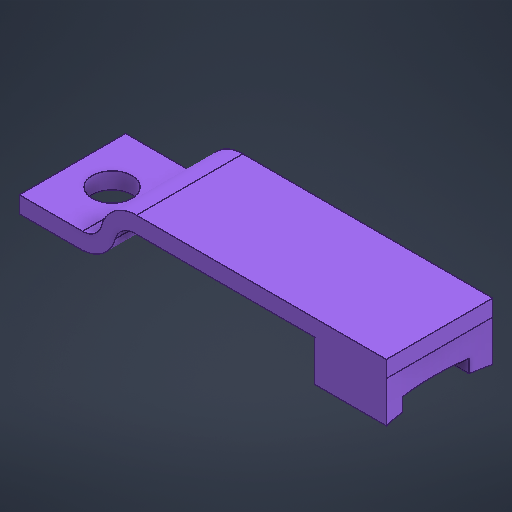
# Autodesk Inventor part: measuring_support1
Saved by Autodesk Inventor 2026.1 (Build 301233000, 233)
## iProperties
Created: 2026-01-06
Part Number: measuring_support1
Material: Generic
Document SubType Name: Modeling
Designer: emanuel
Density: 1 g/cm^3
Appearance: Violet
Author: emanuel
Autodesk Inventor part; units mm, degrees
ref_plane "YZ Plane" through (0, 0, 0) normal (1, 0, 0) x (0, 1, 0)
ref_plane "XZ Plane" through (0, 0, 0) normal (0, 1, 0) x (-1, 0, 0)
ref_plane "XY Plane" through (0, 0, 0) normal (0, 0, 1) x (1, 0, 0)
sketch "Sketch1" plane through (0, 0, 0) normal (0, 1, 0) x (-1, 0, 0)
  circle A0 centre (0, 0) radius 39.95
  circle A1 centre (0, 0) radius 35.05
  line L0 (0, 0) -> (0, -5.05)
  line L1 (0, -5.05) -> (60, -5.05)
  line L2 (60, -5.05) -> (60, 5.05)
  line L3 (60, 5.05) -> (0, 5.05)
  line L4 (0, 5.05) -> (0, -5.05)
  line L5 (0, -5.05) -> (60, -5.05)
  line L6 (60, -5.05) -> (60, -8.05)
  line L7 (60, -8.05) -> (0, -8.05)
  line L8 (0, -8.05) -> (0, -5.05)
  line L9 (0, 5.05) -> (60, 5.05)
  line L10 (60, 5.05) -> (60, 8.05)
  line L11 (60, 8.05) -> (0, 8.05)
  line L12 (0, 8.05) -> (0, 5.05)
  line L13 (39.95, 0) -> (44.95, 0)
  line L14 (44.95, 0) -> (44.95, -8.05)
  line L15 (44.95, 0) -> (44.95, 8.05)
  point P0 (34.113, 8.05)
  point P1 (34.113, -8.05)
  point P2 (44.95, -5.05)
  point P3 (34.6843, -5.05)
  point P4 (34.6843, 5.05)
  point P5 (44.95, 5.05)
  point P6 (39.6295, 5.05)
  point P7 (39.6295, -5.05)
  dimension "d0" = 79.9
  dimension "d1" = 70.1
  dimension "d2" = 5.05
  dimension "d3" = 60
  dimension "d4" = 10.1
  dimension "d5" = 60
  dimension "d6" = 3
  dimension "d7" = 60
  dimension "d8" = 3
  dimension "d9" = 5
  constraints: 32 end point, 6 parallel, 4 horizontal, 4 perpendicular, 3 point on line, 2 coincident, 1 centre point, 1 vertical, 3 other
  measures "d1" diameter of A1
  measures "d2" distance of L0.start L0.end
  measures "d3" distance of L3.end L2.end
  measures "d4" distance of L2.end L1.end
  measures "d5" distance of L6.end L7.end
  measures "d6" distance of L5.end L6.end
  measures "d7" distance of L11.end L10.end
  measures "d8" distance of L10.end L9.end
  measures "d9" distance of L13.start L13.end
extrude "Extrusion1" add sketch "Sketch1" along normal blind 4.2 contours A0 L1 A1 L3 | L13 L14 L1 A0 | A0 L3 L15 L13 | L3 A1 L11 A0 | A0 L11 L15 L3 | L1 L14 L7 A0 | A0 L7 A1 L1
extrude "Extrusion2" add sketch "Sketch1" against normal blind 2 contours L3 A1 L11 A0 | A0 L11 L15 L3 | L1 L14 L7 A0 | A0 L7 A1 L1
extrude "Extrusion3" cut sketch "Sketch1" along normal blind 1 contours L13 L14 L1 A0 | A0 L3 L15 L13
sketch "Sketch4" plane through (-44.95, 4.2, 8.05) normal (0, 0, 1) x (1, 0, 0)
  line L0 (0, 0) -> (10.837, 0) projected
  line L1 (10.837, 0) -> (0, 0)
  line L2 (0, 0) -> (0, 2.5)
  line L3 (0, 2.5) -> (10.837, 2.5)
  line L4 (10.837, 2.5) -> (10.837, 0)
  line L5 (0, 2.5) -> (-30, 2.5)
  line L6 (-30, 2.5) -> (-30, 0)
  line L7 (-30, 0) -> (0, 0)
  line L8 (0, 0) -> (0, 2.5)
  line L9 (-30, 2.5) -> (-32.5, 2.5)
  line L10 (-32.5, 2.5) -> (-32.5, -6.2)
  line L11 (-32.5, -6.2) -> (-30, -6.2)
  line L12 (-30, -6.2) -> (-30, 2.5)
  line L13 (-32.5, -6.2) -> (-44.75, -6.2)
  line L14 (-44.75, -6.2) -> (-44.75, -3.7)
  line L15 (-44.75, -3.7) -> (-32.5, -3.7)
  line L16 (-32.5, -3.7) -> (-32.5, -6.2)
  point P0 (44.95, -4.2)
  point P1 (-30, 0)
  point P2 (-32.5, -3.7)
  dimension "d26" = 2.5
  dimension "d27" = 30
  dimension "d28" = 2.5
  dimension "d29" = 8.7
  dimension "d30" = 2.5
  dimension "d31" = 12.25
  constraints: 32 end point, 8 parallel, 4 horizontal, 4 perpendicular
  measures "d26" distance of L1.end L2.end
  measures "d27" distance of L7.end L6.end
  measures "d28" distance of L11.end L10.end
  measures "d29" distance of L10.end L9.end
  measures "d30" distance of L13.end L14.end
  measures "d31" distance of L14.end L15.end
extrude "Extrusion6" add sketch "Sketch4" against normal up to surface (16.1 mm away)
sketch "Sketch5" plane through (-74.95, 4.2, 8.05) normal (0, -1, 0) x (1, 0, 0)
  line L0 (30, -16.1) -> (30, 0) projected
  line L1 (30, -8.05) -> (-8.75, -8.05)
  circle A0 centre (-8.75, -8.05) radius 3
  point P0 (74.95, -8.05)
  dimension "d34" = 38.75
  dimension "d35" = 6
  constraints: 2 end point, 1 centre point, 1 coincident, 1 horizontal, 1 midpoint
  measures "d34" distance of L1.start L1.end
  measures "d35" diameter of A0
extrude "Extrusion7" cut sketch "Sketch5" along normal blind 10
fillet "Fillet1" radius 5.5 2 edges at (-77.45, 6.7, 0) (-74.95, -2, 0)
fillet "Fillet2" radius 3 2 edges at (-74.95, 4.2, 0) (-77.45, 0.5, 0)
body "Solid1"
